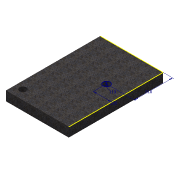
# Autodesk Inventor part: plinth
Saved by Autodesk Inventor 2017 (Build 210142000, 142)
## iProperties
Created: 2014-03-11
Part Number: plinth
Material: Concrete
Document SubType Name: Modeling
Designer: Dave
Density: 2.40731 g/cm^3
Appearance: Exposed Aggregate - Coarse
Mass: 77996.9 g
Surface Area: 17640 cm^2
Volume: 32400 cm^3
Author: Dave
Autodesk Inventor part; units mm, degrees
ref_plane "YZ Plane" through (0, 0, 0) normal (1, 0, 0) x (0, 1, 0)
ref_plane "XZ Plane" through (0, 0, 0) normal (0, 1, 0) x (-1, 0, 0)
ref_plane "XY Plane" through (0, 0, 0) normal (0, 0, 1) x (1, 0, 0)
sketch "Sketch1" plane through (0, 0, 0) normal (0, 1, 0) x (-1, 0, 0)
  line L0 (0, 0) -> (1000, 0)
  line L1 (1000, 0) -> (1000, 1500)
  line L2 (1000, 1500) -> (0, 1500)
  line L3 (0, 1500) -> (0, 0)
  dimension "d0" = 1000
  dimension "d1" = 1500
  constraints: 8 end point, 2 parallel, 1 horizontal, 1 perpendicular
  measures "d0" distance of L2.end L1.end
  measures "d1" distance of L2.end L0.start
extrude "base" add sketch "Sketch1" along normal blind 150
sketch "Sketch2" plane through (0, 150, 0) normal (0, 1, 0) x (1, 0, 0)
  circle A0 centre (-290, -610) radius 55
  line L0 (0, 0) -> (-1000, 0) projected
  line L1 (0, -1500) -> (0, 0) projected
  dimension "d4" = 110
  dimension "d38" = 610
  dimension "d62" = 290
  constraints: 1 centre point
  measures "d4" diameter of A0
  measures "d38" distance from line of A0.centre L0
  measures "d62" distance from line of L1 A0.centre
extrude "air" cut sketch "Sketch2" against normal through all
sketch "Sketch6" plane through (0, 150, 0) normal (0, 1, 0) x (1, 0, 0)
  line L0 (-1000, 0) -> (-1000, -1500) projected
  circle A0 centre (-880, -1350) radius 55
  line L1 (-1000, -1500) -> (0, -1500) projected
  dimension "d56" = 110
  dimension "d60" = 150
  dimension "d61" = 120
  constraints: 1 centre point
  measures "d56" diameter of A0
  measures "d60" distance from line of L1 A0.centre
  measures "d61" distance from line of L0 A0.centre
hole "air2" at (-880, 150, 1350) direction (0, -1, 0) diameter 110 end through all
body "Solid1"
